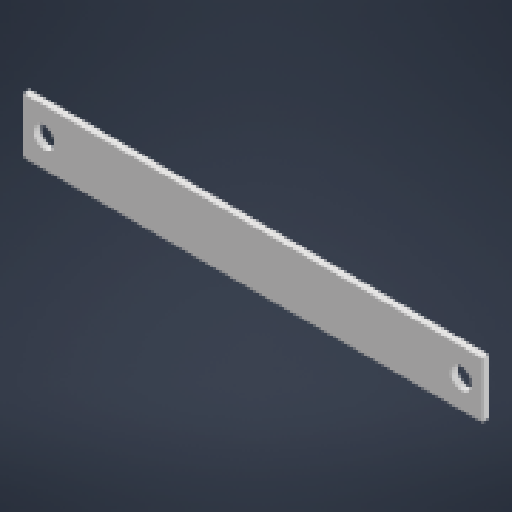
# Autodesk Inventor part: FrameBottomBeam
Saved by Autodesk Inventor 2024 (Build 280153000, 153)
## iProperties
Created: 2025-03-17
Part Number: FrameBottomBeam
Material: Stainless Steel
Document SubType Name: Sheet Metal
Designer: Tommy Rohmann
Density: 8 g/cm^3
Sheet Metal Rule: Default
Appearance: Semi-Polished
Author: Tommy Rohmann
Autodesk Inventor part; units mm, degrees
ref_plane "YZ Plane" through (0, 0, 0) normal (1, 0, 0) x (0, 1, 0)
ref_plane "XZ Plane" through (0, 0, 0) normal (0, 1, 0) x (-1, 0, 0)
ref_plane "XY Plane" through (0, 0, 0) normal (0, 0, 1) x (1, 0, 0)
sketch "FrameBottomBeam" plane through (0, 0, 0) normal (0, 0, 1) x (1, 0, 0)
  line L0 (104.1884, 9.7512) -> (104.1884, -15.6488)
  line L1 (-0.5866, -15.6488) -> (-0.5866, 9.7512)
  line L2 (104.1884, 9.7512) -> (-0.5866, 9.7512)
  line L3 (104.1884, -15.6488) -> (-0.5866, -15.6488)
  line L4 (70.8001, -15.6488) -> (70.8001, 9.7512)
  line L5 (-105.3616, 9.7512) -> (-105.3616, -15.6488)
  line L6 (-105.3616, 9.7512) -> (-0.5866, 9.7512)
  line L7 (-105.3616, -15.6488) -> (-0.5866, -15.6488)
  line L8 (-71.9733, -15.6488) -> (-71.9733, 9.7512)
  circle A0 centre (-95.8366, -2.9488) radius 4.7625
  circle A1 centre (94.6634, -2.9488) radius 4.7625
  point P0 (-8.6642, 25.0995)
  dimension "d227" = 209.55
  dimension "d228" = 142.7734
  dimension "d244" = 25.4
  dimension "d615" = 12.7
  dimension "d616" = 9.525
  dimension "d617" = 9.525
  measures "d227" diameter of L0 L1
  measures "d228" diameter of L4 L1
  measures "d244" distance between parallel lines of L3 L2
  measures "d615" distance from line of A0.centre L6
  measures "d616" diameter of A0
  measures "d617" distance from line of L5 A0.centre
derived "LAYOUT.ipt"
sketch "Sketch1" plane through (0, 0, 0) normal (0, 0, 1) x (1, 0, 0)
  line L0 (104.1884, 9.7512) -> (104.1884, -15.6488)
  line L1 (-0.5866, -15.6488) -> (-0.5866, 9.7512)
  line L2 (104.1884, 9.7512) -> (-0.5866, 9.7512)
  line L3 (104.1884, -15.6488) -> (-0.5866, -15.6488)
  line L4 (70.8001, -15.6488) -> (70.8001, 9.7512)
  line L5 (-105.3616, 9.7512) -> (-105.3616, -15.6488)
  line L6 (-105.3616, 9.7512) -> (-0.5866, 9.7512)
  line L7 (-105.3616, -15.6488) -> (-0.5866, -15.6488)
  line L8 (-71.9733, -15.6488) -> (-71.9733, 9.7512)
  circle A0 centre (-95.8366, -2.9488) radius 4.7625
  circle A1 centre (94.6634, -2.9488) radius 4.7625
extrude "Plate1" add sketch "Sketch1" along normal blind 3.048
equation "\"d1\" = Thickness"
equation "\"BendRadius\" = Thickness"
equation "\"BendReliefWidth\" = Thickness"
equation "\"BendReliefDepth\" = 0.5 * Thickness"
equation "\"CornerReliefSize\" = 4 * Thickness"
equation "\"MinimumRemnant\" = 2 * Thickness"
equation "\"TransitionRadius\" = BendRadius"
equation "\"JacobiRadiusSize\" = BendRadius"
equation "\"GapSize\" = Thickness"
equation "\"Thickness\" = 3.048"
body "Solid1"
